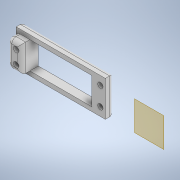
# Autodesk Inventor part: hank joint two bracket
Saved by Autodesk Inventor 2022 (Build 260153000, 153)
## iProperties
Created: 2021-06-27
Part Number: hank joint two bracket
Material: Generic
Document SubType Name: Modeling
Designer: chris
Density: 1 g/cm^3
Appearance: Default
Author: chris
Autodesk Inventor part; units mm, degrees
ref_plane "YZ Plane" through (0, 0, 0) normal (1, 0, 0) x (0, 1, 0)
ref_plane "XZ Plane" through (0, 0, 0) normal (0, 1, 0) x (-1, 0, 0)
ref_plane "XY Plane" through (0, 0, 0) normal (0, 0, 1) x (1, 0, 0)
sketch "Sketch1" plane through (0, 0, 0) normal (0, 0, 1) x (1, 0, 0)
  circle A0 centre (0, 0) radius 15.875
  line L0 (0, 0) -> (-100, 0)
  line L1 (-100, 0) -> (-100, -15.875)
  line L2 (-100, -15.875) -> (0, -15.875)
  line L3 (0, 15.875) -> (-100, 15.875)
  line L4 (-100, 15.875) -> (-100, 0)
  circle A1 centre (-93.65, -4.953) radius 1.9939
  circle A2 centre (-45.0344, 4.953) radius 1.9939
  line L5 (-89.6622, 10.16) -> (-89.6622, -10.16)
  line L6 (-89.6622, 10.16) -> (-49.0222, 10.16)
  line L7 (-49.0222, 10.16) -> (-49.0222, -10.16)
  line L8 (-49.0222, -10.16) -> (-89.6622, -10.16)
  line L9 (-69.3422, 10.16) -> (-69.3422, 4.953)
  circle A3 centre (-45.0344, -4.953) radius 1.9939
  circle A4 centre (-93.65, 4.953) radius 1.9939
  circle A5 centre (-8.001, 0) radius 1
  circle A6 centre (8.001, 0) radius 1
  circle A7 centre (0, 0) radius 1.4986
  line L10 (-43.0405, 10.16) -> (-43.0405, -15.875)
  line L11 (-43.0405, 10.16) -> (-43.0405, 15.875)
  line L12 (-49.0222, 10.16) -> (-43.0405, 10.16)
  line L13 (-49.0222, -10.16) -> (-43.0405, -10.16)
  line L14 (-89.6622, 15.875) -> (-89.6622, -15.875)
  line L15 (-32.9694, 15.875) -> (-32.9694, -15.875)
  point P0 (-89.6622, 0)
  dimension "d0" = 31.75
  dimension "d1" = 100
  dimension "d3" = 6.35
  dimension "d4" = 4.953
  dimension "d5" = 3.9878
  dimension "d6" = 3.9878
  dimension "d7" = 4.953
  dimension "d8" = 20.32
  dimension "d9" = 40.64
  dimension "d10" = 3.9878
  dimension "d11" = 8.001
  dimension "d12" = 2
  dimension "d13" = 2
  dimension "d14" = 8.001
  dimension "d15" = 2.9972
  dimension "d33" = 12.065
  constraints: 32 end point, 9 perpendicular, 9 point on line, 8 centre point, 2 coincident, 2 horizontal, 2 midpoint, 2 point on circle, 2 symmetric about line, 2 vertical, 1 horizontal alignment, 1 parallel, 1 tangent, 1 vertical alignment, 2 other
  measures "d0" diameter of A0
  measures "d1" distance of L0.start L0.end
  measures "d3" distance from line of L1 A1.centre
  measures "d4" distance from line of L0 A1.centre
  measures "d5" diameter of A1
  measures "d6" diameter of A2
  measures "d7" distance from line of L0 A2.centre
  measures "d8" distance of L5.start L5.end
  measures "d9" distance of L5.start L6.end
  measures "d10" distance from line of A1.centre L5
  measures "d11" distance of point (0, 0) A5.centre
  measures "d12" diameter of A5
  measures "d13" diameter of A6
  measures "d14" distance of point (0, 0) A6.centre
  measures "d15" diameter of A7
  measures "d33" distance from line of L15 A2.centre
ref_plane "Work Plane1" through (0, 0, 6.35) normal (0, 0, 1) x (1, 0, 0)
sketch "Sketch3" plane through (0, 0, 6.35) normal (0, 0, 1) x (1, 0, 0)
  circle A0 centre (-93.65, -4.953) radius 1.9939 projected
  line L0 (-89.6622, -10.16) -> (-89.6622, 10.16) projected
  line L1 (-89.6622, 10.16) -> (-43.0405, 10.16) projected
  line L2 (-43.0405, -10.16) -> (-89.6622, -10.16) projected
  line L3 (-43.0405, 10.16) -> (-43.0405, -10.16) projected
  point P0 (0, 0)
ref_plane "Work Plane2" through (0, 0, 6.35) normal (0, 0, 1) x (1, 0, 0)
extrude "Extrusion6" add sketch "Sketch1" along normal blind 6.35 contours L15 L0 L10 L11 L3 | L2 L10 L0 L15 | L11 L12 L6 L14 L3 | L2 L14 L8 L13 L10 | L14 L5 L0 L4 L3 | L2 L1 L0 L5 L14
sketch "Sketch9" plane through (0, 0, 6.35) normal (0, 0, 1) x (1, 0, 0)
  circle A0 centre (-45.0344, 4.953) radius 1.9939 projected
  circle A1 centre (-45.0344, -4.953) radius 1.9939 projected
  line L0 (-32.9694, -15.875) -> (-32.9694, 15.875) projected
  line L1 (-32.9694, 0) -> (52.4257, 0)
  circle A2 centre (-36.6524, 6.9469) radius 1.9939
  circle A3 centre (-36.6524, -6.9469) radius 1.9939
  point P0 (0, 0)
  dimension "d38" = 3.9878
  dimension "d39" = 8.382
  dimension "d40" = 3.9878
  constraints: 2 centre point, 2 end point, 1 horizontal, 1 midpoint
  measures "d38" diameter of A2
  measures "d39" horizontal distance of A0.centre A2.centre
  measures "d40" diameter of A3
extrude "Extrusion7" cut sketch "Sketch9" against normal blind 6.35 contours A2 | A3
sketch "Sketch10" plane through (0, 0, 6.35) normal (0, 0, 1) x (1, 0, 0)
  circle A0 centre (-36.6524, -6.9469) radius 1.9939 projected
  circle A1 centre (-36.6524, 6.9469) radius 1.9939 projected
  line L0 (-32.9694, 15.875) -> (-100, 15.875) projected
  line L1 (-100, 15.875) -> (-100, -15.875) projected
  line L2 (-100, -15.875) -> (-32.9694, -15.875) projected
  line L3 (-32.9694, -15.875) -> (-32.9694, 15.875) projected
  circle A2 centre (-93.65, -4.953) radius 1.9939 projected
  line L4 (-43.0405, 10.16) -> (-43.0405, -10.16) projected
  line L5 (-43.0405, -10.16) -> (-89.6622, -10.16) projected
  line L6 (-89.6622, -10.16) -> (-89.6622, 10.16) projected
  line L7 (-89.6622, 10.16) -> (-43.0405, 10.16) projected
  circle A3 centre (-93.65, 4.953) radius 1.9939 projected
  line L8 (-32.9694, 15.875) -> (-100, 15.875) projected
  line L9 (-89.6622, 15.875) -> (-89.6622, -15.875)
  line L10 (-100, -15.875) -> (-32.9694, -15.875) projected
  point P0 (0, 0)
  constraints: 2 end point, 2 point on line, 1 perpendicular
extrude "Extrusion8" add sketch "Sketch10" along normal blind 6.35 contours L9 L6 L2 L1 L0
sketch "Sketch12" plane through (0, 0, 12.7) normal (0, 0, 1) x (1, 0, 0)
  line L0 (-89.6622, 15.875) -> (-89.6622, 10.16) projected
  line L1 (-89.6622, 10.16) -> (-43.0405, 10.16) projected
  line L2 (-43.0405, 10.16) -> (-43.0405, -10.16) projected
  line L3 (-43.0405, -10.16) -> (-89.6622, -10.16) projected
  line L4 (-89.6622, -10.16) -> (-89.6622, -15.875) projected
  line L5 (-89.6622, -15.875) -> (-32.9694, -15.875) projected
  line L6 (-32.9694, -15.875) -> (-32.9694, 15.875) projected
  line L7 (-32.9694, 15.875) -> (-89.6622, 15.875) projected
  circle A0 centre (-36.6524, -6.9469) radius 1.9939 projected
  circle A1 centre (-36.6524, 6.9469) radius 1.9939 projected
  line L8 (-89.6622, -15.875) -> (-32.9694, -15.875) projected
  line L9 (-89.6622, -15.875) -> (-110.2427, -15.875)
  line L10 (-110.2427, -15.875) -> (-110.2427, -10.16)
  line L11 (-43.0405, -10.16) -> (-89.6622, -10.16) projected
  line L12 (-110.2427, -10.16) -> (-89.6622, -10.16)
  line L13 (-89.6622, 15.875) -> (-89.6622, 10.16) projected
  line L14 (-89.6622, -10.16) -> (-89.6622, 10.16)
  line L15 (-89.6622, 10.16) -> (-117.0886, 10.16)
  line L16 (-117.0886, 10.16) -> (-117.0886, 15.875)
  line L17 (-117.0886, 15.875) -> (-89.6622, 15.875)
  point P0 (0, 0)
  constraints: 14 end point, 5 perpendicular, 1 collinear, 1 point on line
extrude "Extrusion9" cut sketch "Sketch12" against normal up to surface (6.35 mm away) contours L0 L15 L16 L17 | L4 L9 L10 L12
fillet "Fillet4" radius 3.175 3 edges at (-89.6622, 0, 12.7) (-94.8311, -10.16, 12.7) (-94.8311, 10.16, 12.7)
sketch "Sketch14" plane through (-100, 15.875, 0) normal (0, 1, 0) x (1, 0, 0)
  line L0 (67.0306, -6.35) -> (0, -6.35) projected
  line L1 (67.0306, 0) -> (67.0306, -6.35) projected
  line L2 (67.0306, 0) -> (0, 0) projected
  line L3 (0, 0) -> (0, -6.35) projected
  point P0 (100, 0)
extrude "Extrusion10" cut sketch "Sketch14" against normal blind 2.54
mirror "Mirror1" about plane through (0, 0, 0) normal (0, 1, 0) of "Extrusion10"
fillet "Fillet7" radius 3.175 9 edges at (-66.4847, 13.335, 0) (-66.4847, -13.335, 0) (-32.9694, 0, 0) (-100, -9.2301, 11.7701) (-100, -10.16, 7.9375) (-100, 9.2301, 11.7701) (-100, 10.16, 7.9375) (-100, 0, 12.7) (-100, 0, 0)
body "Solid1"
